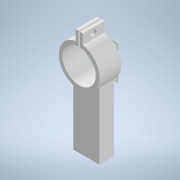
# Autodesk Inventor part: base_motor
Saved by Autodesk Inventor 2022 (Build 260153000, 153)
## iProperties
Created: 2022-03-03
Part Number: base_motor
Material: Generic
Document SubType Name: Modeling
Designer: katha
Density: 1 g/cm^3
Appearance: Default
Author: katha
Autodesk Inventor part; units mm, degrees
ref_plane "YZ Plane" through (0, 0, 0) normal (1, 0, 0) x (0, 1, 0)
ref_plane "XZ Plane" through (0, 0, 0) normal (0, 1, 0) x (-1, 0, 0)
ref_plane "XY Plane" through (0, 0, 0) normal (0, 0, 1) x (1, 0, 0)
ref_plane "Work Plane3" through (158.3589, -41.348, 102.8428) normal (0, 0, -1) x (-1, 0, 0)
sketch "Sketch3" plane through (158.3589, -41.348, 102.8428) normal (0, 0, -1) x (-1, 0, 0)
  circle A0 centre (0, 0) radius 10.5 projected
  arc A1 (-0.5, 11.4891) -> (0.5, 11.4891) centre (0, 0) ccw
  line L0 (0, 0) -> (0, 16.5106) construction
  line L1 (-2.5, 13.775) -> (-2.5, 20.775)
  line L2 (-0.5, 11.4891) -> (-0.5, 20.775)
  line L3 (-2.5, 20.775) -> (-0.5, 20.775)
  line L4 (2.5, 13.775) -> (2.5, 20.775)
  line L5 (0.5, 11.4891) -> (0.5, 20.775)
  line L6 (2.5, 20.775) -> (0.5, 20.775)
  arc A2 (-2.5, 13.775) -> (2.5, 13.775) centre (0, 0) ccw
  point P0 (158.3589, 41.348)
  dimension "d8" = 1
  dimension "d10" = 2.5
  dimension "d11" = 2
  dimension "d12" = 7
  dimension "d13" = 14
  constraints: 14 end point, 4 point on circle, 4 symmetric about line, 3 vertical, 2 centre point, 1 horizontal
  measures "d8" radial gap between concentric circles of A0 A1
  measures "d10" horizontal distance of L0.start L1.start
  measures "d11" distance between parallel lines of L2 L1
  measures "d12" distance of L1.start L1.end
  measures "d13" radius of A2
extrude "Extrusion2" add sketch "Sketch3" against normal blind 15 contours A1 L5 L6 L4 A2 L1 L3 L2
sketch "Sketch4" plane through (160.8589, -27.573, 102.8428) normal (1, 0, 0) x (0, 0, -1)
  line L0 (0, 7) -> (0, 0) projected
  line L1 (0, 7) -> (-15, 7) projected
  line L2 (-15, 0) -> (-15, 7) projected
  line L3 (0, 0) -> (-15, 0) projected
  line L4 (0, 7) -> (-15, 7) projected
  line L5 (-7.5, 7) -> (-7.5, 0) construction
  line L6 (0, 0) -> (-15, 0) projected
  line L7 (-15, 0) -> (-15, 7) projected
  line L8 (-15, 3.5) -> (0, 3.5) construction
  line L9 (0, 7) -> (0, 0) projected
  circle A0 centre (-7.5, 3.5) radius 2.015
  point P0 (102.8428, 27.573)
  dimension "d16" = 4.03
  constraints: 5 midpoint, 4 end point, 1 centre point
  measures "d16" diameter of A0
extrude "Extrusion3" cut sketch "Sketch4" against normal blind 15 contours A0
sketch "Sketch5" plane through (158.3589, -41.348, 102.8428) normal (0, 0, -1) x (-1, 0, 0)
  line L0 (-41.6411, -56.9287) -> (358.3589, -56.9287) projected
  arc A0 (-2.5, 13.775) -> (2.5, 13.775) centre (0, 0) ccw projected
  line L1 (0, -14) -> (0, -56.9287) construction
  line L2 (9, -10.7238) -> (9, -56.9287)
  line L3 (-9, -10.7238) -> (-9, -56.9287)
  point P0 (158.3589, 41.348)
  point P1 (-9, -10.7238)
  point P2 (-9, -56.9287)
  dimension "d19" = 9
  constraints: 6 end point, 2 perpendicular, 2 point on circle, 2 point on line, 2 symmetric about line
  measures "d19" distance between parallel lines of L2 L1
extrude "Extrusion4" add sketch "Sketch5" against normal blind 15
ref_plane "Work Plane5" through (0, -98.2767, 225.7428) normal (0, 1, 0) x (-1, 0, 0)
sketch "Sketch7" plane through (0, -98.2767, 225.7428) normal (0, 1, 0) x (-1, 0, 0)
  circle A0 centre (-143.3589, -112.9) radius 2 projected
  circle A1 centre (-173.3589, -112.9) radius 2 projected
  line L0 (-134.3589, -107.9) -> (-182.3589, -107.9)
  line L1 (-182.3589, -107.9) -> (-182.3589, -122.9)
  line L2 (-182.3589, -122.9) -> (-134.3589, -122.9)
  line L3 (-134.3589, -122.9) -> (-134.3589, -107.9)
  line L4 (-144.3589, -107.9) -> (-155.8589, -107.9) projected
  point P0 (0, -225.7428)
  point P1 (-149.3589, -107.9)
  dimension "d23" = 48
  dimension "d24" = 15
  dimension "d25" = 9
  constraints: 8 end point, 2 parallel, 1 collinear, 1 horizontal, 1 perpendicular
  measures "d23" distance of L2.end L1.end
  measures "d24" distance of L2.end L0.start
  measures "d25" distance from line of L3 A0.centre
extrude "Extrusion5" add sketch "Sketch7" along normal blind 3
body "Solid2"
